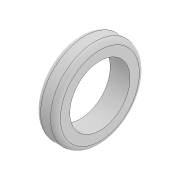
# Autodesk Inventor part: front shaft stopper
Saved by Autodesk Inventor 2022 (Build 260153000, 153)
## iProperties
Created: 2024-08-29
Part Number: front shaft stopper
Material: Generic
Document SubType Name: Modeling
Designer: david
Density: 1 g/cm^3
Appearance: Default
Author: david
Autodesk Inventor part; units mm, degrees
ref_plane "YZ Plane" through (0, 0, 0) normal (1, 0, 0) x (0, 1, 0)
ref_plane "XZ Plane" through (0, 0, 0) normal (0, 1, 0) x (-1, 0, 0)
ref_plane "XY Plane" through (0, 0, 0) normal (0, 0, 1) x (1, 0, 0)
sketch "Sketch1" plane through (0, 0, 0) normal (1, 0, 0) x (0, 1, 0)
  circle A0 centre (0, 0) radius 2.85
  circle A1 centre (0, 0) radius 4.5
  dimension "d0" = 5.7
  dimension "d1" = 9
  constraints: 2 centre point, 2 coincident
  measures "d0" diameter of A0
  measures "d1" diameter of A1
extrude "Extrusion1" add sketch "Sketch1" along normal mid plane 2
fillet "Fillet1" radius 0.5 2 edges at (1, -4.5, 0) (-1, -4.5, 0)
thicken "Thicken4" operation add thickness 0.2 both sides no extend neighbours yes toward (0, 0.9967573, -0.0804666) faces at (0.6667, 2.8408, -0.2293) (-0.6667, 2.8408, -0.2293)
body "Solid1"
